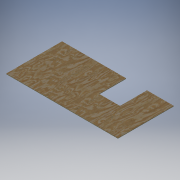
# Autodesk Inventor part: Table Top .25 in
Saved by Autodesk Inventor 2016 (Build 200138000, 138)
## iProperties
Created: 2016-04-01
Part Number: Table Top .25 in
Material: Generic
Document SubType Name: Modeling
Designer: amycroft3
Density: 1 g/cm^3
Appearance: Smooth - Ash
Author: amycroft3
Autodesk Inventor part; units mm, degrees
ref_plane "YZ Plane" through (0, 0, 0) normal (1, 0, 0) x (0, 1, 0)
ref_plane "XZ Plane" through (0, 0, 0) normal (0, 1, 0) x (-1, 0, 0)
ref_plane "XY Plane" through (0, 0, 0) normal (0, 0, 1) x (1, 0, 0)
sketch "Sketch1" plane through (0, 0, 0) normal (0, 1, 0) x (-1, 0, 0)
  line L0 (609.6, 304.8) -> (-609.6, 304.8)
  line L1 (-609.6, 304.8) -> (-609.6, -304.8)
  line L2 (-609.6, -304.8) -> (609.6, -304.8)
  line L3 (609.6, -304.8) -> (609.6, 304.8)
  line L4 (609.6, 304.8) -> (-609.6, -304.8) construction
  line L5 (-609.6, 304.8) -> (609.6, -304.8) construction
  point P0 (0, 0)
  dimension "d0" = 609.6
  dimension "d1" = 1219.2
  constraints: 12 end point, 2 midpoint, 2 parallel, 1 horizontal, 1 perpendicular
  measures "d0" distance of L2.end L0.start
  measures "d1" distance of L0.start L0.end
extrude "Extrusion1" add sketch "Sketch1" along normal blind 6.35
sketch "Sketch2" plane through (0, 6.35, 0) normal (0, 1, 0) x (1, 0, 0)
  line L0 (88.9, 10.16) -> (317.5, 10.16)
  line L1 (317.5, 10.16) -> (317.5, 304.8)
  line L2 (317.5, 304.8) -> (88.9, 304.8)
  line L3 (88.9, 304.8) -> (88.9, 10.16)
  line L4 (88.9, 10.16) -> (317.5, 304.8) construction
  line L5 (317.5, 10.16) -> (88.9, 304.8) construction
  line L6 (609.6, 304.8) -> (-609.6, 304.8) projected
  line L7 (-609.6, 304.8) -> (-609.6, -304.8) projected
  line L8 (609.6, -304.8) -> (609.6, 304.8) projected
  point P0 (0, 0)
  point P1 (203.2, 157.48)
  dimension "d4" = 228.6
  dimension "d5" = 294.64
  dimension "d9" = 292.1
  constraints: 12 end point, 2 midpoint, 2 parallel, 1 collinear, 1 horizontal, 1 perpendicular
  measures "d4" distance of L1.end L2.end
  measures "d5" distance of L0.end L1.end
  measures "d9" distance between parallel lines of L1 L8
extrude "Extrusion2" cut sketch "Sketch2" against normal up to next
sketch "Sketch3" plane through (0, 6.35, 0) normal (0, 1, 0) x (1, 0, 0)
  circle A0 centre (298.45, -262.1026) radius 2.54
  circle A1 centre (298.45, -234.1626) radius 2.54
  circle A2 centre (82.55, -262.1026) radius 2.54
  circle A3 centre (82.55, -234.1626) radius 2.54
  line L0 (-609.6, -304.8) -> (609.6, -304.8) projected
  line L1 (609.6, -304.8) -> (609.6, 304.8) projected
  line L2 (317.5, 304.8) -> (317.5, 10.16) projected
  circle A4 centre (217.17, -2.54) radius 2.54
  circle A5 centre (189.23, -2.54) radius 2.54
  line L3 (317.5, 10.16) -> (88.9, 10.16) projected
  line L4 (88.9, 10.16) -> (88.9, 304.8) projected
  line L5 (88.9, 10.16) -> (317.5, 10.16) projected
  line L6 (203.2, 10.16) -> (203.2, -2.54) construction
  point P0 (0, 0)
  dimension "d10" = 5.08
  dimension "d14" = 27.94
  dimension "d16" = 215.9
  dimension "d18" = 42.6974
  dimension "d26" = 19.05
  dimension "d27" = 12.7
  dimension "d31" = 27.94
  constraints: 6 centre point, 5 equal radius, 4 horizontal alignment, 2 end point, 2 vertical alignment, 1 midpoint, 1 symmetric about line, 1 vertical
  measures "d10" diameter of A0
  measures "d14" distance of A1.centre A0.centre
  measures "d16" distance of A2.centre A0.centre
  measures "d18" distance from line of L0 A0.centre
  measures "d26" distance from line of A0.centre L2
  measures "d27" distance from line of A4.centre L3
  measures "d31" distance of A5.centre A4.centre
extrude "Extrusion4" cut sketch "Sketch3" against normal up to next
body "Solid1"
